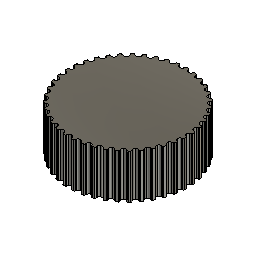
gear_43z (Autodesk Fusion 360 design; units mm, degrees)
Autodesk Fusion 360 part; units mm, degrees
sketch "Sketch1" plane through (0, 0, 0) normal (0, 0, 1) x (1, 0, 0) in component "gt2 pulley"
  circle A0 centre (0, 0) radius 13.6873 construction
  circle A1 centre (0, 0) radius 12.6833 construction
  line L0 (0, 0) -> (0, 13.6873) construction
  line L1 (0, 0) -> (0.9991, 13.6508) construction
  line L2 (0, 0) -> (1.4081, 13.6147) construction
  circle A2 centre (0, 0) radius 13.4333 construction
  arc A3 (0.3844, 13.2918) -> (0.448, 13.0047) centre (1.3819, 13.3621) ccw
  circle A4 centre (0, 0) radius 13.2833 construction
  arc A5 (0.2374, 13.4312) -> (0, 13.4333) centre (0, 0) ccw
  arc A6 (0.3844, 13.2918) -> (0.2374, 13.4312) centre (0.2348, 13.2812) ccw
  arc A7 (0.448, 13.0047) -> (0.9258, 12.6495) centre (0.9663, 13.203) ccw
  arc A8 (0, 13.4333) -> (-0.2374, 13.4312) centre (0, 0) ccw
  arc A9 (-0.2374, 13.4312) -> (-0.3844, 13.2918) centre (-0.2348, 13.2812) ccw
  arc A10 (-0.448, 13.0047) -> (-0.3844, 13.2918) centre (-1.3819, 13.3621) ccw
  arc A11 (-0.9258, 12.6495) -> (-0.448, 13.0047) centre (-0.9663, 13.203) ccw
  arc A12 (0.9258, 12.6495) -> (-0.9258, 12.6495) centre (0, 0) ccw
  point P0 (1.3819, 13.3621)
  point P1 (0, 13.4333)
  dimension "d18" = 27.3747
  dimension "d19" = 4.186
  dimension "d22" = 1.004
  dimension "d24" = 0.75
  dimension "d26" = 1
  dimension "d27" = 0.15
  dimension "d28" = 0.15
  dimension "d47" = 0.555
  dimension "d52" = 3.812
  constraint coincident A0.centre A1.centre
  constraint coincident A0 L0.end
  constraint vertical L0
  constraint coincident A0 L1.end
  constraint coincident A0 L2.end
  constraint concentric A1 A2
  constraint coincident A1 A7.end
  constraint coincident L1 A7.end
  constraint coincident A2 P0
  constraint coincident L2 P0
  constraint coincident P0 A3.centre
  constraint coincident A2 P1
  constraint coincident L0 P1
  constraint concentric A2 A4
  constraint coincident P1 A5.end
  constraint coincident A4 A6.centre
  constraint coincident A3.start A6.start
  constraint tangent A3 A6
  constraint tangent A3 A7
  constraint symmetric L0 A7.end A11.start
  constraint symmetric L0 A3.start A9.end
  constraint symmetric L0 A3.end A10.start
  constraint symmetric L0 A3 A10
  constraint symmetric L0 A5.start A8.end
  constraint symmetric L0 P1 A5.end
  constraint symmetric L0 A5 A8
  constraint symmetric L0 A6 A9
  constraint symmetric L0 A7 A11
  constraint coincident A1 A11.start
  constraint tangent A1 A7
  constraint coincident L1 A7.centre
  measures "d18" diameter of A0
  measures "d19" angle of L0 L1
  measures "d22" distance of A0 A1
  measures "d24" distance of A1 A2
  measures "d26" radius of A3
  measures "d27" distance of A2 A4
  measures "d28" radius of A6
  measures "d47" radius of A7
extrude "Extrude1" add sketch "Sketch1" along normal blind 10 makes body 1
pattern_circular "C-Pattern1" count 43 over 360 about axis through (0, 0, 1.75) along (0, 0, 1) of bodies 1 makes body 2 at (-1.336, 12.6128, 6.6667) makes body 3 at (-4.338, 11.9184, 6.6667) makes body 4 at (-4.7226, 11.7713, 3.3333) makes body 5 at (-7.5877, 10.1633, 6.6667) makes body 6 at (-8.5402, 9.3772, 6.6667) makes body 7 at (-9.8145, 8.0338, 6.6667) makes body 8 at (-10.8797, 6.5191, 6.6667) makes body 9 at (-11.7129, 4.8656, 6.6667) makes body 10 at (-12.2966, 3.1083, 6.6667) makes body 11 at (-12.6181, 1.2848, 6.6667) makes body 12 at (-12.6807, 0.2574, 3.3333) makes body 13 at (-12.3214, -3.0084, 6.6667) makes body 14 at (-11.752, -4.7704, 6.6667) makes body 15 at (-11.591, -5.1494, 3.3333) makes body 16 at (-9.8794, -7.9538, 6.6667) makes body 17 at (-9.059, -8.877, 6.6667) makes body 18 at (-8.3093, -9.5824, 3.3333) makes body 19 at (-6.8256, -10.6901, 3.3333) makes body 20 at (-3.8507, -12.0846, 6.6667) makes body 21 at (-3.4564, -12.2033, 3.3333) makes body 22 at (-0.8231, -12.6566, 6.6667) makes body 23 at (0.2059, -12.6817, 3.3333) makes body 24 at (2.0502, -12.5165, 3.3333) makes body 25 at (4.6269, -11.8093, 6.6667) makes body 26 at (6.8256, -10.6901, 6.6667) makes body 27 at (7.1691, -10.4629, 3.3333) makes body 28 at (9.616, -8.2704, 6.6667) makes body 29 at (10.3748, -7.2959, 6.6667) makes body 30 at (11.591, -5.1494, 6.6667) makes body 31 at (11.752, -4.7703, 3.3333) makes body 32 at (12.4906, -2.2024, 6.6667) makes body 33 at (12.6782, -0.3603, 6.6667) makes body 34 at (12.5956, 1.4895, 6.6667) makes body 35 at (12.2445, 3.3076, 6.6667) makes body 36 at (11.9359, 4.2895, 3.3333) makes body 37 at (10.7724, 6.6949, 6.6667) makes body 38 at (9.2725, 8.6538, 6.6667) makes body 39 at (7.9137, 9.9116, 6.6667) makes body 40 at (6.9121, 10.6343, 6.6667) makes body 41 at (6.0271, 11.1598, 3.3333) makes body 42 at (2.9583, 12.3335, 6.6667) makes body 43 at (2.5564, 12.423, 3.3333)
sketch "Sketch2" plane through (0, 0, 10) normal (0, 0, 1) x (-1, 0, 0)
  arc A0 (-5.9899, -11.8719) -> (-5.9159, -12.0605) centre (-5.8499, -11.9258) ccw
  arc A1 (-5.9159, -12.0605) -> (-5.486, -12.262) centre (0, 0) ccw
  arc A2 (-5.486, -12.262) -> (-5.2937, -12.1982) centre (-5.4247, -12.1251) ccw
  arc A3 (-5.1143, -11.9652) -> (-5.2937, -12.1982) centre (-4.4203, -12.6852) ccw
  arc A4 (-4.5309, -11.8464) -> (-5.1143, -11.9652) centre (-4.7291, -12.3648) ccw
  arc A5 (-6.2074, -11.0605) -> (-4.5309, -11.8464) centre (0, 0) ccw
  arc A6 (-5.9255, -11.5849) -> (-6.2074, -11.0605) centre (-6.4791, -11.5445) ccw
  arc A7 (-5.9899, -11.8719) -> (-5.9255, -11.5849) centre (-6.9229, -11.5121) ccw
  circle A8 centre (0, 0) radius 12.6833
  constraint coincident A1.centre A5.centre
extrude "Extrude2" add sketch "Sketch2" against normal blind 10 contours A5 A8 bodies 1 2 3 4 5 6 7 8 9 10 11 12 13 14 15 16 17 18 19 20 21 22 23 24 25 26 27 28 29 30 31 32 33 34 35 36 37 38 39 40 41 42 43
extrude "Extrude4" [suppressed] in component "gt2 pulley"
pattern_circular "C-Pattern7" [suppressed] in component "gt2 pulley"
extrude "Extrude3" [suppressed] in component "gt2 pulley"
pattern_circular "C-Pattern6" [suppressed] in component "gt2 pulley"
extrude "Extrude2'" [suppressed] in component "gt2 pulley"
pattern_circular "C-Pattern5" [suppressed] in component "gt2 pulley"
extrude "Extrude1'" [suppressed] in component "gt2 pulley"
pattern_circular "C-Pattern4" [suppressed] in component "gt2 pulley"
pattern_circular "C-Pattern3" [suppressed] in component "gt2 pulley"
pattern_circular "C-Pattern2" [suppressed] in component "gt2 pulley"
pattern_circular "C-Pattern1'" [suppressed] in component "gt2 pulley"
copy_body "Body->Comp1" [suppressed] in component "Component"
copy_body "Body->Comp2" [suppressed] in component "Component'"
copy_body "Body->Comp3" [suppressed] in component "Component''"
copy_body "Body->Comp4" [suppressed] in component "Component'''"
copy_body "Body->Comp5" [suppressed] in component "Component''''"
copy_body "Body->Comp6" [suppressed] in component "Component'''''"
copy_body "Body->Comp7" [suppressed] in component "Component''''''"
copy_body "Body->Comp8" [suppressed] in component "Component'''''''"
copy_body "Body->Comp9" [suppressed] in component "Component''''''''"
copy_body "Body->Comp10" [suppressed] in component "Component'''''''''"
copy_body "Body->Comp11" [suppressed] in component "Component''''''''''"
copy_body "Body->Comp12" [suppressed] in component "Component'''''''''''"
copy_body "Body->Comp13" [suppressed] in component "Component''''''''''''"
copy_body "Body->Comp14" [suppressed] in component "Component'''''''''''''"
copy_body "Body->Comp15" [suppressed] in component "Component''''''''''''''"
copy_body "Body->Comp16" [suppressed] in component "Component'''''''''''''''"
copy_body "Body->Comp17" [suppressed] in component "Component''''''''''''''''"
copy_body "Body->Comp18" [suppressed] in component "Component'''''''''''''''''"
copy_body "Body->Comp19" [suppressed] in component "Component''''''''''''''''''"
copy_body "Body->Comp20" [suppressed] in component "Component'''''''''''''''''''"
component "gt2 pulley" placed x (1, 0, 0) y (0, 1, 0) z (0, 0, 1) at (0, 0, 0)
equation "NumTeeth = 43" comment "min 20"
equation "ToothPitch = 2 mm"
equation "PullyDia = NumTeeth * ToothPitch / PI"
equation "ToothAng = ( ( 360 / NumTeeth ) * 1 deg )"
equation "TransOffsetAngle = ToothAng * 0.2"
equation "Sholulder_Radius = 0.15 mm"
equation "Root_Radius = 0.555 mm"
equation "TransRadius = 1 mm"
equation "ToolHeight = 0.75 mm"
equation "PLD = 0.254 mm"
equation "d18 = PullyDia"
equation "d19 = ToothAng / 2"
equation "d22 = PLD + ToolHeight"
equation "d24 = ToolHeight"
equation "d26 = TransRadius"
equation "d27 = Sholulder_Radius"
equation "d31 = NumTeeth"
equation "d33 = NumTeeth"
equation "d35 = NumTeeth"
equation "d37 = NumTeeth"
equation "d41 = NumTeeth"
equation "d45 = NumTeeth"
equation "d47 = Root_Radius"
equation "d50 = NumTeeth"
